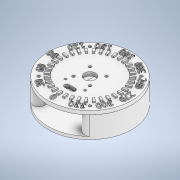
# Autodesk Inventor part: dual_motor_testbed_cover
Saved by Autodesk Inventor 2022.2 (Build 262287000, 287)
## iProperties
Created: 2018-11-22
Part Number: dual_motor_testbed_cover
Material: Generic
Document SubType Name: Modeling
Designer: Jochen
Density: 1 g/cm^3
Appearance: Default
Sending System: SolidWorks 2017
Last Author: Felix
Last Saved: 2021-02-24
Author: Jochen
Autodesk Inventor part; units mm, degrees
(part 1 of 2)
ref_plane "YZ Plane" through (0, 0, 0) normal (1, 0, 0) x (0, 1, 0)
ref_plane "XZ Plane" through (0, 0, 0) normal (0, 1, 0) x (-1, 0, 0)
ref_plane "XY Plane" through (0, 0, 0) normal (0, 0, 1) x (1, 0, 0)
sketch "Sketch1" plane through (0, 0, 0) normal (0, 1, 0) x (-1, 0, 0)
  line L0 (0, -76.3335) -> (0, 76.0077) construction
  line L1 (124.8346, 0) -> (-26.138, 0) construction
  circle A0 centre (50, 0) radius 6
  circle A1 centre (50, 0) radius 12.5 construction
  line L2 (46.5, 21.5) -> (53.5, 21.5)
  line L3 (46.5, 19) -> (53.5, 19)
  line L4 (53.5, 24) -> (46.5, 24)
  arc A2 (46.5, 24) -> (46.5, 19) centre (46.5, 21.5) ccw
  arc A3 (53.5, 19) -> (53.5, 24) centre (53.5, 21.5) ccw
  circle A4 centre (60.48, 15.75) radius 1.25
  circle A5 centre (39.52, 15.75) radius 1.25
  circle A6 centre (58.8388, 8.8388) radius 1.5
  circle A7 centre (58.8388, -8.8388) radius 1.5
  circle A8 centre (41.1612, -8.8388) radius 1.5
  circle A9 centre (41.1612, 8.8388) radius 1.5
  line L5 (58.8388, 8.8388) -> (41.1612, 8.8388) construction
  line L6 (41.1612, 8.8388) -> (41.1612, -8.8388) construction
  line L7 (41.1612, -8.8388) -> (58.8388, -8.8388) construction
  line L8 (58.8388, -8.8388) -> (58.8388, 8.8388) construction
  line L9 (50, 8.8388) -> (50, -8.8388) construction
  line L10 (51, 35) -> (49, 35)
  line L11 (49, 35) -> (49, 30)
  line L12 (49, 30) -> (51, 30)
  line L13 (51, 30) -> (51, 35)
  line L14 (85.5155, 3.449) -> (91.318, 3.449) construction
  line L15 (91.318, 3.449) -> (91.318, 5.2094) construction
  line L16 (91.318, 5.2094) -> (85.5155, 5.2094) construction
  line L17 (85.5155, 5.2094) -> (85.5155, 3.449) construction
  line L18 (43.3702, -36.2504) -> (56.0342, -36.2504) construction
  line L19 (56.0342, -36.2504) -> (56.0342, -42.8053) construction
  line L20 (56.0342, -42.8053) -> (43.3702, -42.8053) construction
  line L21 (43.3702, -42.8053) -> (43.3702, -36.2504) construction
  line L22 (9.6343, 14.1663) -> (13.2809, 21.7068) construction
  line L23 (13.2809, 21.7068) -> (20.1891, 18.366) construction
  line L24 (20.1891, 18.366) -> (16.5425, 10.8255) construction
  line L25 (16.5425, 10.8255) -> (9.6343, 14.1663) construction
  line L26 (65, 35.5829) -> (65, 35.8735) construction
  line L27 (52.3586, 36.3581) -> (47.6414, 36.3581) construction
  line L28 (47.6414, 36.3581) -> (47.6414, 35) construction
  line L29 (47.6414, 35) -> (52.3586, 35) construction
  line L30 (52.3586, 35) -> (52.3586, 36.3581) construction
  line L31 (45.7754, 29.7179) -> (44.9071, 34.6419)
  line L32 (44.9071, 34.6419) -> (42.9375, 34.2946)
  line L33 (42.9375, 34.2946) -> (43.8057, 29.3706)
  line L34 (43.8057, 29.3706) -> (45.7754, 29.7179)
  line L35 (40.6791, 28.5328) -> (38.969, 33.2313)
  line L36 (38.969, 33.2313) -> (37.0896, 32.5472)
  line L37 (37.0896, 32.5472) -> (38.7997, 27.8488)
  line L38 (38.7997, 27.8488) -> (40.6791, 28.5328)
  line L39 (35.866, 26.4808) -> (33.366, 30.8109)
  line L40 (33.366, 30.8109) -> (31.634, 29.8109)
  line L41 (31.634, 29.8109) -> (34.134, 25.4808)
  line L42 (34.134, 25.4808) -> (35.866, 26.4808)
  line L43 (31.4824, 23.6241) -> (28.2685, 27.4543)
  line L44 (28.2685, 27.4543) -> (26.7364, 26.1688)
  line L45 (26.7364, 26.1688) -> (29.9503, 22.3385)
  line L46 (29.9503, 22.3385) -> (31.4824, 23.6241)
  line L47 (27.6615, 20.0497) -> (23.8312, 23.2636)
  line L48 (23.8312, 23.2636) -> (22.5457, 21.7315)
  line L49 (22.5457, 21.7315) -> (26.3759, 18.5176)
  line L50 (26.3759, 18.5176) -> (27.6615, 20.0497)
  line L51 (24.5192, 15.866) -> (20.1891, 18.366)
  line L52 (20.1891, 18.366) -> (19.1891, 16.634)
  line L53 (19.1891, 16.634) -> (23.5192, 14.134)
  line L54 (23.5192, 14.134) -> (24.5192, 15.866)
  line L55 (22.1512, 11.2003) -> (17.4528, 12.9104)
  line L56 (17.4528, 12.9104) -> (16.7687, 11.031)
  line L57 (16.7687, 11.031) -> (21.4672, 9.3209)
  line L58 (21.4672, 9.3209) -> (22.1512, 11.2003)
  line L59 (20.6294, 6.1943) -> (15.7054, 7.0625)
  line L60 (15.7054, 7.0625) -> (15.3581, 5.0929)
  line L61 (15.3581, 5.0929) -> (20.2821, 4.2246)
  line L62 (20.2821, 4.2246) -> (20.6294, 6.1943)
  line L63 (20, 1) -> (15, 1)
  line L64 (15, 1) -> (15, -1)
  line L65 (15, -1) -> (20, -1)
  line L66 (20, -1) -> (20, 1)
  line L67 (20.2821, -4.2246) -> (15.3581, -5.0929)
  line L68 (15.3581, -5.0929) -> (15.7054, -7.0625)
  line L69 (15.7054, -7.0625) -> (20.6294, -6.1943)
  line L70 (20.6294, -6.1943) -> (20.2821, -4.2246)
  line L71 (21.4672, -9.3209) -> (16.7687, -11.031)
  line L72 (16.7687, -11.031) -> (17.4528, -12.9104)
  line L73 (17.4528, -12.9104) -> (22.1512, -11.2003)
  line L74 (22.1512, -11.2003) -> (21.4672, -9.3209)
  line L75 (23.5192, -14.134) -> (19.1891, -16.634)
  line L76 (19.1891, -16.634) -> (20.1891, -18.366)
  line L77 (20.1891, -18.366) -> (24.5192, -15.866)
  line L78 (24.5192, -15.866) -> (23.5192, -14.134)
  line L79 (26.3759, -18.5176) -> (22.5457, -21.7315)
  line L80 (22.5457, -21.7315) -> (23.8312, -23.2636)
  line L81 (23.8312, -23.2636) -> (27.6615, -20.0497)
  line L82 (27.6615, -20.0497) -> (26.3759, -18.5176)
  line L83 (29.9503, -22.3385) -> (26.7364, -26.1688)
  line L84 (26.7364, -26.1688) -> (28.2685, -27.4543)
  line L85 (28.2685, -27.4543) -> (31.4824, -23.6241)
  line L86 (31.4824, -23.6241) -> (29.9503, -22.3385)
  line L87 (34.134, -25.4808) -> (31.634, -29.8109)
  line L88 (31.634, -29.8109) -> (33.366, -30.8109)
  line L89 (33.366, -30.8109) -> (35.866, -26.4808)
  line L90 (35.866, -26.4808) -> (34.134, -25.4808)
  line L91 (38.7997, -27.8488) -> (37.0896, -32.5472)
  line L92 (37.0896, -32.5472) -> (38.969, -33.2313)
  line L93 (38.969, -33.2313) -> (40.6791, -28.5328)
  line L94 (40.6791, -28.5328) -> (38.7997, -27.8488)
  line L95 (43.8057, -29.3706) -> (42.9375, -34.2946)
  line L96 (42.9375, -34.2946) -> (44.9071, -34.6419)
  line L97 (44.9071, -34.6419) -> (45.7754, -29.7179)
  line L98 (45.7754, -29.7179) -> (43.8057, -29.3706)
  line L99 (49, -30) -> (49, -35)
  line L100 (49, -35) -> (51, -35)
  line L101 (51, -35) -> (51, -30)
  line L102 (51, -30) -> (49, -30)
  line L103 (54.2246, -29.7179) -> (55.0929, -34.6419)
  line L104 (55.0929, -34.6419) -> (57.0625, -34.2946)
  line L105 (57.0625, -34.2946) -> (56.1943, -29.3706)
  line L106 (56.1943, -29.3706) -> (54.2246, -29.7179)
  line L107 (59.3209, -28.5328) -> (61.031, -33.2313)
  line L108 (61.031, -33.2313) -> (62.9104, -32.5472)
  line L109 (62.9104, -32.5472) -> (61.2003, -27.8488)
  line L110 (61.2003, -27.8488) -> (59.3209, -28.5328)
  line L111 (64.134, -26.4808) -> (66.634, -30.8109)
  line L112 (66.634, -30.8109) -> (68.366, -29.8109)
  line L113 (68.366, -29.8109) -> (65.866, -25.4808)
  line L114 (65.866, -25.4808) -> (64.134, -26.4808)
  line L115 (68.5176, -23.6241) -> (71.7315, -27.4543)
  line L116 (71.7315, -27.4543) -> (73.2636, -26.1688)
  line L117 (73.2636, -26.1688) -> (70.0497, -22.3385)
  line L118 (70.0497, -22.3385) -> (68.5176, -23.6241)
  line L119 (72.3385, -20.0497) -> (76.1688, -23.2636)
  line L120 (76.1688, -23.2636) -> (77.4543, -21.7315)
  line L121 (77.4543, -21.7315) -> (73.6241, -18.5176)
  line L122 (73.6241, -18.5176) -> (72.3385, -20.0497)
  line L123 (75.4808, -15.866) -> (79.8109, -18.366)
  line L124 (79.8109, -18.366) -> (80.8109, -16.634)
  line L125 (80.8109, -16.634) -> (76.4808, -14.134)
  line L126 (76.4808, -14.134) -> (75.4808, -15.866)
  line L127 (77.8488, -11.2003) -> (82.5472, -12.9104)
  line L128 (82.5472, -12.9104) -> (83.2313, -11.031)
  line L129 (83.2313, -11.031) -> (78.5328, -9.3209)
  line L130 (78.5328, -9.3209) -> (77.8488, -11.2003)
  line L131 (79.3706, -6.1943) -> (84.2946, -7.0625)
  line L132 (84.2946, -7.0625) -> (84.6419, -5.0929)
  line L133 (84.6419, -5.0929) -> (79.7179, -4.2246)
  line L134 (79.7179, -4.2246) -> (79.3706, -6.1943)
  line L135 (80, -1) -> (85, -1)
  line L136 (85, -1) -> (85, 1)
  line L137 (85, 1) -> (80, 1)
  line L138 (80, 1) -> (80, -1)
  line L139 (79.7179, 4.2246) -> (84.6419, 5.0929)
  line L140 (84.6419, 5.0929) -> (84.2946, 7.0625)
  line L141 (84.2946, 7.0625) -> (79.3706, 6.1943)
  line L142 (79.3706, 6.1943) -> (79.7179, 4.2246)
  line L143 (78.5328, 9.3209) -> (83.2313, 11.031)
  line L144 (83.2313, 11.031) -> (82.5472, 12.9104)
  line L145 (82.5472, 12.9104) -> (77.8488, 11.2003)
  line L146 (77.8488, 11.2003) -> (78.5328, 9.3209)
  line L147 (76.4808, 14.134) -> (80.8109, 16.634)
  line L148 (80.8109, 16.634) -> (79.8109, 18.366)
  line L149 (79.8109, 18.366) -> (75.4808, 15.866)
  line L150 (75.4808, 15.866) -> (76.4808, 14.134)
  line L151 (73.6241, 18.5176) -> (77.4543, 21.7315)
  line L152 (77.4543, 21.7315) -> (76.1688, 23.2636)
  line L153 (76.1688, 23.2636) -> (72.3385, 20.0497)
  line L154 (72.3385, 20.0497) -> (73.6241, 18.5176)
  line L155 (70.0497, 22.3385) -> (73.2636, 26.1688)
  line L156 (73.2636, 26.1688) -> (71.7315, 27.4543)
  line L157 (71.7315, 27.4543) -> (68.5176, 23.6241)
  line L158 (68.5176, 23.6241) -> (70.0497, 22.3385)
  line L159 (65.866, 25.4808) -> (68.366, 29.8109)
  line L160 (68.366, 29.8109) -> (66.634, 30.8109)
  line L161 (66.634, 30.8109) -> (64.134, 26.4808)
  line L162 (64.134, 26.4808) -> (65.866, 25.4808)
  line L163 (61.2003, 27.8488) -> (62.9104, 32.5472)
  line L164 (62.9104, 32.5472) -> (61.031, 33.2313)
  line L165 (61.031, 33.2313) -> (59.3209, 28.5328)
  line L166 (59.3209, 28.5328) -> (61.2003, 27.8488)
  line L167 (56.1943, 29.3706) -> (57.0625, 34.2946)
  line L168 (57.0625, 34.2946) -> (55.0929, 34.6419)
  line L169 (55.0929, 34.6419) -> (54.2246, 29.7179)
  line L170 (54.2246, 29.7179) -> (56.1943, 29.3706)
  arc A10 (95, 0) -> (10.2941, 21.1765) centre (50, 0) ccw
  arc A11 (10.2941, 21.1765) -> (95, 0) centre (50, 0) ccw
  circle A12 centre (77.5, 27.5) radius 1.5
  circle A13 centre (77.5, -27.5) radius 1.5
  circle A14 centre (22.5, -27.5) radius 1.5
  circle A15 centre (22.5, 27.5) radius 1.5
  line L171 (77.5, 27.5) -> (22.5, 27.5) construction
  line L172 (22.5, 27.5) -> (22.5, -27.5) construction
  line L173 (22.5, -27.5) -> (77.5, -27.5) construction
  line L174 (77.5, -27.5) -> (77.5, 27.5) construction
  line L175 (71.3909, 27.5) -> (71.3909, -27.5)
  arc A16 (71.3909, -27.5) -> (81.8198, -31.8198) centre (77.5, -27.5) ccw
  arc A17 (18.1802, -31.8198) -> (28.6091, -27.5) centre (22.5, -27.5) ccw
  arc A18 (81.8198, 31.8198) -> (71.3909, 27.5) centre (77.5, 27.5) ccw
  arc A19 (28.6091, 27.5) -> (18.1802, 31.8198) centre (22.5, 27.5) ccw
  line L176 (28.6091, 27.5) -> (28.6091, -27.5)
  line L177 (7.333, -7.0802) -> (7.333, 0) construction
  line L178 (7.333, 0) -> (17.5306, 0) construction
  line L179 (17.5306, 0) -> (17.5306, -7.0802) construction
  line L180 (17.5306, -7.0802) -> (7.333, -7.0802) construction
  line L181 (22.3605, 33.283) -> (34.2819, 40.1658) construction
  line L182 (34.2819, 40.1658) -> (31.501, 44.9824) construction
  line L183 (31.501, 44.9824) -> (19.5797, 38.0996) construction
  line L184 (19.5797, 38.0996) -> (22.3605, 33.283) construction
  line L185 (16.4835, -27.645) -> (12.2955, -20.3911) construction
  line L186 (12.2955, -20.3911) -> (18.941, -16.5543) construction
  line L187 (18.941, -16.5543) -> (23.129, -23.8082) construction
  line L188 (23.129, -23.8082) -> (16.4835, -27.645) construction
  line L189 (25.9985, -27.8884) -> (33.1783, -32.0337) construction
  line L190 (33.1783, -32.0337) -> (25.8889, -44.6591) construction
  line L191 (25.8889, -44.6591) -> (18.7092, -40.5139) construction
  line L192 (18.7092, -40.5139) -> (25.9985, -27.8884) construction
  line L193 (69.3835, -47.2114) -> (62.0942, -34.5859) construction
  line L194 (62.0942, -34.5859) -> (69.2739, -30.4407) construction
  line L195 (69.2739, -30.4407) -> (76.5632, -43.0661) construction
  line L196 (76.5632, -43.0661) -> (69.3835, -47.2114) construction
  line L197 (90.9137, -31.4796) -> (78.2883, -24.1903) construction
  line L198 (78.2883, -24.1903) -> (82.4335, -17.0105) construction
  line L199 (82.4335, -17.0105) -> (95.059, -24.2998) construction
  line L200 (95.059, -24.2998) -> (90.9137, -31.4796) construction
  line L201 (70.6585, 43.5756) -> (67.8777, 38.759) construction
  line L202 (67.8777, 38.759) -> (79.799, 31.8762) construction
  line L203 (79.799, 31.8762) -> (82.5798, 36.6928) construction
  line L204 (82.5798, 36.6928) -> (70.6585, 43.5756) construction
  line L205 (89.2101, 27.3822) -> (84.3935, 24.6014) construction
  line L206 (84.3935, 24.6014) -> (91.2763, 12.68) construction
  line L207 (91.2763, 12.68) -> (96.0929, 15.4608) construction
  line L208 (96.0929, 15.4608) -> (89.2101, 27.3822) construction
  spline S0 degree 2 poles (11.181, 15.741) (11.0842, 15.5407) (10.9905, 15.0973) (10.9737, 14.8694) knots 0 0 0 1 2 2 2
  spline S1 degree 2 poles (10.9737, 14.8694) (10.9632, 14.6548) (10.9965, 14.3147) (11.0182, 14.1779) knots 0 0 0 1 2 2 2
  line L209 (11.0182, 14.1779) -> (10.9966, 14.1334)
  line L210 (10.9966, 14.1334) -> (10.2179, 14.5101)
  spline S2 degree 2 poles (10.2179, 14.5101) (10.205, 14.8128) (10.394, 15.7372) (10.5726, 16.1066) knots 0 0 0 1 2 2 2
  spline S3 degree 2 poles (10.5726, 16.1066) (10.7534, 16.4804) (11.1737, 16.9635) (11.4437, 17.113) knots 0 0 0 1 2 2 2
  spline S4 degree 2 poles (11.4437, 17.113) (11.7335, 17.2694) (12.3569, 17.2754) (12.6951, 17.1118) knots 0 0 0 1 2 2 2
  spline S5 degree 2 poles (12.6951, 17.1118) (13.149, 16.8923) (13.5459, 15.9645) (13.4326, 15.5032) knots 0 0 0 1 2 2 2
  line L211 (13.4326, 15.5032) -> (13.486, 15.4774)
  spline S6 degree 2 poles (13.486, 15.4774) (13.6056, 15.6337) (13.9573, 15.9523) (14.1993, 16.0439) knots 0 0 0 1 2 2 2
  spline S7 degree 2 poles (14.1993, 16.0439) (14.4369, 16.1377) (15.0386, 16.1103) (15.399, 15.9359) knots 0 0 0 1 2 2 2
  spline S8 degree 2 poles (15.399, 15.9359) (15.7684, 15.7573) (16.2732, 15.2002) (16.4016, 14.8526) knots 0 0 0 1 2 2 2
  spline S9 degree 2 poles (16.4016, 14.8526) (16.5346, 14.4917) (16.4634, 13.686) (16.2547, 13.2544) knots 0 0 0 1 2 2 2
  spline S10 degree 2 poles (16.2547, 13.2544) (16.0545, 12.8405) (15.4626, 12.1274) (15.1912, 11.9182) knots 0 0 0 1 2 2 2
  line L212 (15.1912, 11.9182) -> (14.4124, 12.2948)
  line L213 (14.4124, 12.2948) -> (14.4382, 12.3482)
  spline S11 degree 2 poles (14.4382, 12.3482) (14.7193, 12.4979) (15.4096, 13.1305) (15.5968, 13.5176) knots 0 0 0 1 2 2 2
  spline S12 degree 2 poles (15.5968, 13.5176) (15.7065, 13.7446) (15.7837, 14.2674) (15.6922, 14.4983) knots 0 0 0 1 2 2 2
  spline S13 degree 2 poles (15.6922, 14.4983) (15.5985, 14.7248) (15.2822, 15.0699) (14.9841, 15.2141) knots 0 0 0 1 2 2 2
  spline S14 degree 2 poles (14.9841, 15.2141) (14.6859, 15.3583) (14.2148, 15.372) (14.0282, 15.2701) knots 0 0 0 1 2 2 2
  spline S15 degree 2 poles (14.0282, 15.2701) (13.8417, 15.1681) (13.5527, 14.7862) (13.4321, 14.537) knots 0 0 0 1 2 2 2
  line L214 (13.4321, 14.537) -> (13.2815, 14.2255)
  line L215 (13.2815, 14.2255) -> (12.6718, 14.5203)
  line L216 (12.6718, 14.5203) -> (12.7902, 14.7651)
  spline S16 degree 2 poles (12.7902, 14.7651) (13.0291, 15.2591) (12.8586, 16.1102) (12.4092, 16.3276) knots 0 0 0 1 2 2 2
  spline S17 degree 2 poles (12.4092, 16.3276) (12.2, 16.4287) (11.8244, 16.4127) (11.673, 16.3267) knots 0 0 0 1 2 2 2
  spline S18 degree 2 poles (11.673, 16.3267) (11.5128, 16.234) (11.2736, 15.9323) (11.181, 15.741) knots 0 0 0 1 2 2 2
  spline S19 degree 2 poles (16.3352, 20.7216) (17.8126, 20.0071) (18.7813, 18.4789) (18.3487, 17.5844) knots 0 0 0 1 2 2 2
  spline S20 degree 2 poles (18.3487, 17.5844) (17.9097, 16.6766) (16.0879, 16.5088) (14.6416, 17.2083) knots 0 0 0 1 2 2 2
  spline S21 degree 2 poles (14.6416, 17.2083) (13.1552, 17.9271) (12.1955, 19.451) (12.6302, 20.3499) knots 0 0 0 1 2 2 2
  spline S22 degree 2 poles (12.6302, 20.3499) (13.0671, 21.2533) (14.9022, 21.4146) (16.3352, 20.7216) knots 0 0 0 1 2 2 2
  spline S23 degree 2 poles (17.5522, 18.969) (17.3324, 19.2071) (16.5388, 19.7007) (15.9736, 19.974) knots 0 0 0 1 2 2 2
  spline S24 degree 2 poles (15.9736, 19.974) (15.4084, 20.2473) (14.5332, 20.5608) (14.1991, 20.5851) knots 0 0 0 1 2 2 2
  spline S25 degree 2 poles (14.1991, 20.5851) (13.8649, 20.6094) (13.3884, 20.3621) (13.2399, 20.0551) knots 0 0 0 1 2 2 2
  spline S26 degree 2 poles (13.2399, 20.0551) (13.0914, 19.748) (13.1891, 19.2121) (13.4224, 18.9565) knots 0 0 0 1 2 2 2
  spline S27 degree 2 poles (13.4224, 18.9565) (13.649, 18.7096) (14.4647, 18.2163) (15.0032, 17.9559) knots 0 0 0 1 2 2 2
  spline S28 degree 2 poles (15.0032, 17.9559) (15.5817, 17.6761) (16.3904, 17.3728) (16.749, 17.3422) knots 0 0 0 1 2 2 2
  spline S29 degree 2 poles (16.749, 17.3422) (17.0855, 17.3113) (17.5841, 17.5588) (17.739, 17.8793) knots 0 0 0 1 2 2 2
  spline S30 degree 2 poles (17.739, 17.8793) (17.8854, 18.1819) (17.7877, 18.7178) (17.5522, 18.969) knots 0 0 0 1 2 2 2
  spline S31 degree 2 poles (18.3281, 24.8425) (19.8055, 24.128) (20.7742, 22.5998) (20.3416, 21.7053) knots 0 0 0 1 2 2 2
  spline S32 degree 2 poles (20.3416, 21.7053) (19.9026, 20.7975) (18.0808, 20.6297) (16.6345, 21.3291) knots 0 0 0 1 2 2 2
  spline S33 degree 2 poles (16.6345, 21.3291) (15.1481, 22.048) (14.1884, 23.5719) (14.6231, 24.4708) knots 0 0 0 1 2 2 2
  spline S34 degree 2 poles (14.6231, 24.4708) (15.06, 25.3742) (16.8951, 25.5355) (18.3281, 24.8425) knots 0 0 0 1 2 2 2
  spline S35 degree 2 poles (19.5451, 23.0899) (19.3253, 23.3279) (18.5317, 23.8215) (17.9665, 24.0949) knots 0 0 0 1 2 2 2
  spline S36 degree 2 poles (17.9665, 24.0949) (17.4013, 24.3682) (16.5261, 24.6816) (16.1919, 24.706) knots 0 0 0 1 2 2 2
  spline S37 degree 2 poles (16.1919, 24.706) (15.8578, 24.7303) (15.3813, 24.483) (15.2328, 24.176) knots 0 0 0 1 2 2 2
  spline S38 degree 2 poles (15.2328, 24.176) (15.0843, 23.8689) (15.182, 23.3329) (15.4153, 23.0773) knots 0 0 0 1 2 2 2
  spline S39 degree 2 poles (15.4153, 23.0773) (15.6419, 22.8305) (16.4576, 22.3372) (16.996, 22.0768) knots 0 0 0 1 2 2 2
  spline S40 degree 2 poles (16.996, 22.0768) (17.5746, 21.797) (18.3833, 21.4937) (18.7419, 21.4631) knots 0 0 0 1 2 2 2
  spline S41 degree 2 poles (18.7419, 21.4631) (19.0784, 21.4322) (19.577, 21.6797) (19.7319, 22.0001) knots 0 0 0 1 2 2 2
  spline S42 degree 2 poles (19.7319, 22.0001) (19.8783, 22.3028) (19.7805, 22.8387) (19.5451, 23.0899) knots 0 0 0 1 2 2 2
  line L217 (47.2705, -42.4888) -> (44.2946, -42.4888)
  line L218 (44.2946, -42.4888) -> (44.2946, -41.866)
  line L219 (44.2946, -41.866) -> (45.4019, -41.866)
  line L220 (45.4019, -41.866) -> (45.4019, -37.7779)
  line L221 (45.4019, -37.7779) -> (44.2946, -37.7779)
  line L222 (44.2946, -37.7779) -> (44.2946, -37.2193)
  spline S43 degree 2 poles (44.2946, -37.2193) (44.9224, -37.2193) (45.5156, -36.8634) (45.5552, -36.3691) knots 0 0 0 1 2 2 2
  line L223 (45.5552, -36.3691) -> (46.1879, -36.3691)
  line L224 (46.1879, -36.3691) -> (46.1879, -41.866)
  line L225 (46.1879, -41.866) -> (47.2705, -41.866)
  line L226 (47.2705, -41.866) -> (47.2705, -42.4888)
  spline S44 degree 2 poles (50.2365, -42.6272) (49.7817, -42.6272) (49.0352, -42.3554) (48.7732, -42.1033) knots 0 0 0 1 2 2 2
  spline S45 degree 2 poles (48.7732, -42.1033) (48.5162, -41.8561) (48.2493, -41.1838) (48.2493, -40.8032) knots 0 0 0 1 2 2 2
  spline S46 degree 2 poles (48.2493, -40.8032) (48.2493, -40.3089) (48.7782, -39.4784) (49.2824, -39.2312) knots 0 0 0 1 2 2 2
  line L227 (49.2824, -39.2312) -> (49.2824, -39.2065)
  spline S47 degree 2 poles (49.2824, -39.2065) (48.8326, -38.9445) (48.3976, -38.3217) (48.3976, -37.857) knots 0 0 0 1 2 2 2
  spline S48 degree 2 poles (48.3976, -37.857) (48.3976, -37.1699) (49.4356, -36.2504) (50.2365, -36.2504) knots 0 0 0 1 2 2 2
  spline S49 degree 2 poles (50.2365, -36.2504) (51.0669, -36.2504) (52.0704, -37.1204) (52.0704, -37.8026) knots 0 0 0 1 2 2 2
  spline S50 degree 2 poles (52.0704, -37.8026) (52.0704, -38.2129) (51.5909, -39.0137) (51.1411, -39.2411) knots 0 0 0 1 2 2 2
  line L228 (51.1411, -39.2411) -> (51.1411, -39.2658)
  spline S51 degree 2 poles (51.1411, -39.2658) (51.6749, -39.513) (52.2237, -40.2248) (52.2237, -40.7883) knots 0 0 0 1 2 2 2
  spline S52 degree 2 poles (52.2237, -40.7883) (52.2237, -41.5694) (51.0867, -42.6272) (50.2365, -42.6272) knots 0 0 0 1 2 2 2
  spline S53 degree 2 poles (51.3833, -40.8674) (51.3833, -40.4918) (51.0867, -40.0469) (50.6665, -39.8195) knots 0 0 0 1 2 2 2
  spline S54 degree 2 poles (50.6665, -39.8195) (50.5281, -39.7404) (50.0634, -39.5575) (49.7718, -39.4388) knots 0 0 0 1 2 2 2
  spline S55 degree 2 poles (49.7718, -39.4388) (49.4356, -39.6613) (49.0748, -40.3237) (49.0748, -40.7439) knots 0 0 0 1 2 2 2
  spline S56 degree 2 poles (49.0748, -40.7439) (49.0748, -41.2975) (49.7421, -42.0192) (50.2463, -42.0192) knots 0 0 0 1 2 2 2
  spline S57 degree 2 poles (50.2463, -42.0192) (50.7604, -42.0192) (51.3833, -41.4013) (51.3833, -40.8674) knots 0 0 0 1 2 2 2
  spline S58 degree 2 poles (51.2696, -37.8125) (51.2696, -37.4022) (50.7209, -36.8535) (50.2315, -36.8535) knots 0 0 0 1 2 2 2
  spline S59 degree 2 poles (50.2315, -36.8535) (49.7866, -36.8535) (49.2181, -37.3429) (49.2181, -37.7631) knots 0 0 0 1 2 2 2
  spline S60 degree 2 poles (49.2181, -37.7631) (49.2181, -38.0646) (49.5098, -38.4848) (49.8014, -38.6529) knots 0 0 0 1 2 2 2
  spline S61 degree 2 poles (49.8014, -38.6529) (49.925, -38.7221) (50.449, -38.9643) (50.6616, -39.0335) knots 0 0 0 1 2 2 2
  spline S62 degree 2 poles (50.6616, -39.0335) (51.0175, -38.7616) (51.2696, -38.1832) (51.2696, -37.8125) knots 0 0 0 1 2 2 2
  spline S63 degree 2 poles (56.7665, -39.4388) (56.7665, -41.08) (55.8125, -42.6174) (54.8189, -42.6174) knots 0 0 0 1 2 2 2
  spline S64 degree 2 poles (54.8189, -42.6174) (53.8104, -42.6174) (52.8663, -41.0503) (52.8663, -39.4438) knots 0 0 0 1 2 2 2
  spline S65 degree 2 poles (52.8663, -39.4438) (52.8663, -37.7927) (53.8203, -36.2653) (54.8189, -36.2653) knots 0 0 0 1 2 2 2
  spline S66 degree 2 poles (54.8189, -36.2653) (55.8224, -36.2653) (56.7665, -37.8471) (56.7665, -39.4388) knots 0 0 0 1 2 2 2
  spline S67 degree 2 poles (55.7185, -41.2975) (55.8372, -40.996) (55.9361, -40.0666) (55.9361, -39.4388) knots 0 0 0 1 2 2 2
  spline S68 degree 2 poles (55.9361, -39.4388) (55.9361, -38.811) (55.8372, -37.8866) (55.7136, -37.5752) knots 0 0 0 1 2 2 2
  spline S69 degree 2 poles (55.7136, -37.5752) (55.59, -37.2638) (55.16, -36.9425) (54.8189, -36.9425) knots 0 0 0 1 2 2 2
  spline S70 degree 2 poles (54.8189, -36.9425) (54.4778, -36.9425) (54.0378, -37.2638) (53.9093, -37.5851) knots 0 0 0 1 2 2 2
  spline S71 degree 2 poles (53.9093, -37.5851) (53.7857, -37.8965) (53.6967, -38.8456) (53.6967, -39.4438) knots 0 0 0 1 2 2 2
  spline S72 degree 2 poles (53.6967, -39.4438) (53.6967, -40.0864) (53.7758, -40.9465) (53.9044, -41.2827) knots 0 0 0 1 2 2 2
  spline S73 degree 2 poles (53.9044, -41.2827) (54.023, -41.599) (54.463, -41.9401) (54.8189, -41.9401) knots 0 0 0 1 2 2 2
  spline S74 degree 2 poles (54.8189, -41.9401) (55.155, -41.9401) (55.595, -41.6188) (55.7185, -41.2975) knots 0 0 0 1 2 2 2
  spline S75 degree 2 poles (85.7923, 1.3431) (85.7923, 1.8128) (86.0988, 2.5938) (86.3658, 2.8756) knots 0 0 0 1 2 2 2
  spline S76 degree 2 poles (86.3658, 2.8756) (86.6179, 3.1474) (87.3544, 3.449) (87.7301, 3.449) knots 0 0 0 1 2 2 2
  spline S77 degree 2 poles (87.7301, 3.449) (88.1503, 3.449) (88.8325, 3.1672) (89.0846, 2.9003) knots 0 0 0 1 2 2 2
  spline S78 degree 2 poles (89.0846, 2.9003) (89.4009, 2.5641) (89.747, 1.4766) (89.747, 0.6412) knots 0 0 0 1 2 2 2
  spline S79 degree 2 poles (89.747, 0.6412) (89.747, -0.1151) (89.4059, -1.4696) (89.0747, -1.9194) knots 0 0 0 1 2 2 2
  spline S80 degree 2 poles (89.0747, -1.9194) (88.7237, -2.394) (87.735, -2.8932) (87.0133, -2.8932) knots 0 0 0 1 2 2 2
  spline S81 degree 2 poles (87.0133, -2.8932) (86.8502, -2.8932) (86.4795, -2.8586) (86.3213, -2.8092) knots 0 0 0 1 2 2 2
  line L229 (86.3213, -2.8092) -> (86.3213, -2.0232)
  line L230 (86.3213, -2.0232) -> (86.3608, -2.0232)
  spline S82 degree 2 poles (86.3608, -2.0232) (86.4646, -2.0825) (86.8996, -2.1864) (87.1221, -2.1864) knots 0 0 0 1 2 2 2
  spline S83 degree 2 poles (87.1221, -2.1864) (87.9229, -2.1864) (88.8374, -1.1285) (88.9017, -0.1497) knots 0 0 0 1 2 2 2
  spline S84 degree 2 poles (88.9017, -0.1497) (88.5754, -0.3722) (87.9822, -0.5749) (87.6312, -0.5749) knots 0 0 0 1 2 2 2
  spline S85 degree 2 poles (87.6312, -0.5749) (87.2951, -0.5749) (86.7365, -0.4266) (86.4547, -0.214) knots 0 0 0 1 2 2 2
  spline S86 degree 2 poles (86.4547, -0.214) (86.1285, 0.0381) (85.7923, 0.8043) (85.7923, 1.3431) knots 0 0 0 1 2 2 2
  spline S87 degree 2 poles (88.9214, 0.8241) (88.9214, 1.442) (88.694, 2.223) (88.4914, 2.4356) knots 0 0 0 1 2 2 2
  spline S88 degree 2 poles (88.4914, 2.4356) (88.3134, 2.6333) (87.9427, 2.7816) (87.7252, 2.7816) knots 0 0 0 1 2 2 2
  spline S89 degree 2 poles (87.7252, 2.7816) (87.2209, 2.7816) (86.6228, 2.0599) (86.6228, 1.3777) knots 0 0 0 1 2 2 2
  spline S90 degree 2 poles (86.6228, 1.3777) (86.6228, 0.9922) (86.8205, 0.4929) (87.038, 0.3149) knots 0 0 0 1 2 2 2
  spline S91 degree 2 poles (87.038, 0.3149) (87.1962, 0.1864) (87.5867, 0.1024) (87.8141, 0.1024) knots 0 0 0 1 2 2 2
  spline S92 degree 2 poles (87.8141, 0.1024) (88.0761, 0.1024) (88.6792, 0.2853) (88.9066, 0.4385) knots 0 0 0 1 2 2 2
  spline S93 degree 2 poles (88.9066, 0.4385) (88.9115, 0.4978) (88.9214, 0.7005) (88.9214, 0.8241) knots 0 0 0 1 2 2 2
  spline S94 degree 2 poles (94.3343, 0.2754) (94.3343, -1.3658) (93.3803, -2.9031) (92.3867, -2.9031) knots 0 0 0 1 2 2 2
  spline S95 degree 2 poles (92.3867, -2.9031) (91.3782, -2.9031) (90.4341, -1.3361) (90.4341, 0.2704) knots 0 0 0 1 2 2 2
  spline S96 degree 2 poles (90.4341, 0.2704) (90.4341, 1.9215) (91.3881, 3.449) (92.3867, 3.449) knots 0 0 0 1 2 2 2
  spline S97 degree 2 poles (92.3867, 3.449) (93.3902, 3.449) (94.3343, 1.8671) (94.3343, 0.2754) knots 0 0 0 1 2 2 2
  spline S98 degree 2 poles (93.2863, -1.5833) (93.405, -1.2817) (93.5038, -0.3524) (93.5038, 0.2754) knots 0 0 0 1 2 2 2
  spline S99 degree 2 poles (93.5038, 0.2754) (93.5038, 0.9032) (93.405, 1.8276) (93.2814, 2.139) knots 0 0 0 1 2 2 2
  spline S100 degree 2 poles (93.2814, 2.139) (93.1578, 2.4504) (92.7278, 2.7717) (92.3867, 2.7717) knots 0 0 0 1 2 2 2
  spline S101 degree 2 poles (92.3867, 2.7717) (92.0456, 2.7717) (91.6056, 2.4504) (91.4771, 2.1291) knots 0 0 0 1 2 2 2
  spline S102 degree 2 poles (91.4771, 2.1291) (91.3535, 1.8177) (91.2645, 0.8686) (91.2645, 0.2704) knots 0 0 0 1 2 2 2
  spline S103 degree 2 poles (91.2645, 0.2704) (91.2645, -0.3722) (91.3436, -1.2323) (91.4722, -1.5684) knots 0 0 0 1 2 2 2
  spline S104 degree 2 poles (91.4722, -1.5684) (91.5908, -1.8848) (92.0308, -2.2259) (92.3867, -2.2259) knots 0 0 0 1 2 2 2
  spline S105 degree 2 poles (92.3867, -2.2259) (92.7228, -2.2259) (93.1628, -1.9046) (93.2863, -1.5833) knots 0 0 0 1 2 2 2
  spline S106 degree 2 poles (48.1173, 39.5317) (48.1173, 41.1729) (49.0714, 42.7103) (50.065, 42.7103) knots 0 0 0 1 2 2 2
  spline S107 degree 2 poles (50.065, 42.7103) (51.0734, 42.7103) (52.0175, 41.1432) (52.0175, 39.5367) knots 0 0 0 1 2 2 2
  spline S108 degree 2 poles (52.0175, 39.5367) (52.0175, 37.8856) (51.0635, 36.3581) (50.065, 36.3581) knots 0 0 0 1 2 2 2
  spline S109 degree 2 poles (50.065, 36.3581) (49.0615, 36.3581) (48.1173, 37.94) (48.1173, 39.5317) knots 0 0 0 1 2 2 2
  spline S110 degree 2 poles (49.1653, 41.3904) (49.0466, 41.0889) (48.9478, 40.1595) (48.9478, 39.5317) knots 0 0 0 1 2 2 2
  spline S111 degree 2 poles (48.9478, 39.5317) (48.9478, 38.9039) (49.0466, 37.9795) (49.1702, 37.6681) knots 0 0 0 1 2 2 2
  spline S112 degree 2 poles (49.1702, 37.6681) (49.2938, 37.3567) (49.7239, 37.0354) (50.065, 37.0354) knots 0 0 0 1 2 2 2
  spline S113 degree 2 poles (50.065, 37.0354) (50.406, 37.0354) (50.846, 37.3567) (50.9745, 37.678) knots 0 0 0 1 2 2 2
  spline S114 degree 2 poles (50.9745, 37.678) (51.0981, 37.9894) (51.1871, 38.9385) (51.1871, 39.5367) knots 0 0 0 1 2 2 2
  spline S115 degree 2 poles (51.1871, 39.5367) (51.1871, 40.1793) (51.108, 41.0394) (50.9795, 41.3756) knots 0 0 0 1 2 2 2
  spline S116 degree 2 poles (50.9795, 41.3756) (50.8608, 41.6919) (50.4209, 42.033) (50.065, 42.033) knots 0 0 0 1 2 2 2
  spline S117 degree 2 poles (50.065, 42.033) (49.7288, 42.033) (49.2889, 41.7117) (49.1653, 41.3904) knots 0 0 0 1 2 2 2
  spline S118 degree 2 poles (24.5248, 33.7164) (24.3322, 33.6051) (24.0056, 33.291) (23.8635, 33.1119) knots 0 0 0 1 2 2 2
  spline S119 degree 2 poles (23.8635, 33.1119) (23.7343, 32.9403) (23.5707, 32.6403) (23.5118, 32.515) knots 0 0 0 1 2 2 2
  line L231 (23.5118, 32.515) -> (23.469, 32.4903)
  line L232 (23.469, 32.4903) -> (23.0364, 33.2394)
  spline S120 degree 2 poles (23.0364, 33.2394) (23.1959, 33.4971) (23.8717, 34.1555) (24.2271, 34.3607) knots 0 0 0 1 2 2 2
  spline S121 degree 2 poles (24.2271, 34.3607) (24.5867, 34.5683) (25.2058, 34.7317) (25.5131, 34.7036) knots 0 0 0 1 2 2 2
  spline S122 degree 2 poles (25.5131, 34.7036) (25.8407, 34.6701) (26.3597, 34.3248) (26.5476, 33.9994) knots 0 0 0 1 2 2 2
  spline S123 degree 2 poles (26.5476, 33.9994) (26.7997, 33.5628) (26.6067, 32.5723) (26.2537, 32.2543) knots 0 0 0 1 2 2 2
  line L233 (26.2537, 32.2543) -> (26.2833, 32.203)
  spline S124 degree 2 poles (26.2833, 32.203) (26.4701, 32.2651) (26.9401, 32.331) (27.1917, 32.2708) knots 0 0 0 1 2 2 2
  spline S125 degree 2 poles (27.1917, 32.2708) (27.4409, 32.2149) (27.9232, 31.854) (28.1234, 31.5073) knots 0 0 0 1 2 2 2
  spline S126 degree 2 poles (28.1234, 31.5073) (28.3286, 31.152) (28.433, 30.4075) (28.3439, 30.0478) knots 0 0 0 1 2 2 2
  spline S127 degree 2 poles (28.3439, 30.0478) (28.2511, 29.6745) (27.7395, 29.0481) (27.3242, 28.8083) knots 0 0 0 1 2 2 2
  spline S128 degree 2 poles (27.3242, 28.8083) (26.9261, 28.5785) (26.0357, 28.3213) (25.6937, 28.3008) knots 0 0 0 1 2 2 2
  line L234 (25.6937, 28.3008) -> (25.2612, 29.0499)
  line L235 (25.2612, 29.0499) -> (25.3125, 29.0796)
  spline S129 degree 2 poles (25.3125, 29.0796) (25.6291, 29.0454) (26.5555, 29.1808) (26.928, 29.3958) knots 0 0 0 1 2 2 2
  spline S130 degree 2 poles (26.928, 29.3958) (27.1463, 29.5219) (27.5039, 29.911) (27.558, 30.1534) knots 0 0 0 1 2 2 2
  spline S131 degree 2 poles (27.558, 30.1534) (27.6078, 30.3934) (27.5401, 30.8566) (27.3745, 31.1434) knots 0 0 0 1 2 2 2
  spline S132 degree 2 poles (27.3745, 31.1434) (27.2089, 31.4302) (26.827, 31.7063) (26.6153, 31.7268) knots 0 0 0 1 2 2 2
  spline S133 degree 2 poles (26.6153, 31.7268) (26.4037, 31.7473) (25.95, 31.5939) (25.7103, 31.4555) knots 0 0 0 1 2 2 2
  line L236 (25.7103, 31.4555) -> (25.4106, 31.2824)
  line L237 (25.4106, 31.2824) -> (25.072, 31.8689)
  line L238 (25.072, 31.8689) -> (25.3075, 32.0049)
  spline S134 degree 2 poles (25.3075, 32.0049) (25.7827, 32.2792) (26.12, 33.079) (25.8704, 33.5114) knots 0 0 0 1 2 2 2
  spline S135 degree 2 poles (25.8704, 33.5114) (25.7542, 33.7126) (25.4345, 33.9105) (25.2609, 33.9244) knots 0 0 0 1 2 2 2
  spline S136 degree 2 poles (25.2609, 33.9244) (25.0763, 33.9377) (24.7089, 33.8226) (24.5248, 33.7164) knots 0 0 0 1 2 2 2
  spline S137 degree 2 poles (28.4891, 36.0051) (28.2964, 35.8939) (27.9698, 35.5797) (27.8277, 35.4007) knots 0 0 0 1 2 2 2
  spline S138 degree 2 poles (27.8277, 35.4007) (27.6985, 35.229) (27.5349, 34.9291) (27.476, 34.8037) knots 0 0 0 1 2 2 2
  line L239 (27.476, 34.8037) -> (27.4332, 34.779)
  line L240 (27.4332, 34.779) -> (27.0006, 35.5282)
  spline S139 degree 2 poles (27.0006, 35.5282) (27.1601, 35.7858) (27.8359, 36.4443) (28.1913, 36.6494) knots 0 0 0 1 2 2 2
  spline S140 degree 2 poles (28.1913, 36.6494) (28.5509, 36.857) (29.17, 37.0204) (29.4773, 36.9924) knots 0 0 0 1 2 2 2
  spline S141 degree 2 poles (29.4773, 36.9924) (29.8049, 36.9589) (30.3239, 36.6135) (30.5118, 36.2882) knots 0 0 0 1 2 2 2
  spline S142 degree 2 poles (30.5118, 36.2882) (30.7639, 35.8515) (30.5709, 34.861) (30.2179, 34.5431) knots 0 0 0 1 2 2 2
  line L241 (30.2179, 34.5431) -> (30.2475, 34.4917)
  spline S143 degree 2 poles (30.2475, 34.4917) (30.4343, 34.5539) (30.9043, 34.6197) (31.1559, 34.5595) knots 0 0 0 1 2 2 2
  spline S144 degree 2 poles (31.1559, 34.5595) (31.4051, 34.5036) (31.8874, 34.1428) (32.0876, 33.796) knots 0 0 0 1 2 2 2
  spline S145 degree 2 poles (32.0876, 33.796) (32.2928, 33.4407) (32.3972, 32.6962) (32.3081, 32.3365) knots 0 0 0 1 2 2 2
  spline S146 degree 2 poles (32.3081, 32.3365) (32.2153, 31.9633) (31.7037, 31.3368) (31.2884, 31.0971) knots 0 0 0 1 2 2 2
  spline S147 degree 2 poles (31.2884, 31.0971) (30.8903, 30.8672) (29.9999, 30.61) (29.6579, 30.5895) knots 0 0 0 1 2 2 2
  line L242 (29.6579, 30.5895) -> (29.2254, 31.3387)
  line L243 (29.2254, 31.3387) -> (29.2767, 31.3683)
  spline S148 degree 2 poles (29.2767, 31.3683) (29.5933, 31.3342) (30.5197, 31.4695) (30.8922, 31.6845) knots 0 0 0 1 2 2 2
  spline S149 degree 2 poles (30.8922, 31.6845) (31.1105, 31.8106) (31.4681, 32.1997) (31.5222, 32.4421) knots 0 0 0 1 2 2 2
  spline S150 degree 2 poles (31.5222, 32.4421) (31.572, 32.6821) (31.5044, 33.1453) (31.3388, 33.4322) knots 0 0 0 1 2 2 2
  spline S151 degree 2 poles (31.3388, 33.4322) (31.1732, 33.719) (30.7912, 33.995) (30.5795, 34.0156) knots 0 0 0 1 2 2 2
  spline S152 degree 2 poles (30.5795, 34.0156) (30.3679, 34.0361) (29.9143, 33.8826) (29.6745, 33.7442) knots 0 0 0 1 2 2 2
  line L244 (29.6745, 33.7442) -> (29.3748, 33.5712)
  line L245 (29.3748, 33.5712) -> (29.0362, 34.1577)
  line L246 (29.0362, 34.1577) -> (29.2717, 34.2936)
  spline S153 degree 2 poles (29.2717, 34.2936) (29.7469, 34.568) (30.0842, 35.3678) (29.8346, 35.8002) knots 0 0 0 1 2 2 2
  spline S154 degree 2 poles (29.8346, 35.8002) (29.7184, 36.0014) (29.3987, 36.1992) (29.2251, 36.2132) knots 0 0 0 1 2 2 2
  spline S155 degree 2 poles (29.2251, 36.2132) (29.0405, 36.2264) (28.6731, 36.1114) (28.4891, 36.0051) knots 0 0 0 1 2 2 2
  spline S156 degree 2 poles (35.5513, 37.2285) (36.3719, 35.8072) (36.3143, 33.9988) (35.4539, 33.502) knots 0 0 0 1 2 2 2
  spline S157 degree 2 poles (35.4539, 33.502) (34.5805, 32.9978) (32.9794, 33.8828) (32.1761, 35.2741) knots 0 0 0 1 2 2 2
  spline S158 degree 2 poles (32.1761, 35.2741) (31.3505, 36.7039) (31.413, 38.5038) (32.2778, 39.0031) knots 0 0 0 1 2 2 2
  spline S159 degree 2 poles (32.2778, 39.0031) (33.1469, 39.5048) (34.7554, 38.607) (35.5513, 37.2285) knots 0 0 0 1 2 2 2
  spline S160 degree 2 poles (35.5731, 35.0948) (35.525, 35.4153) (35.146, 36.2696) (34.8321, 36.8133) knots 0 0 0 1 2 2 2
  spline S161 degree 2 poles (34.8321, 36.8133) (34.5182, 37.3569) (33.9704, 38.1081) (33.7077, 38.316) knots 0 0 0 1 2 2 2
  spline S162 degree 2 poles (33.7077, 38.316) (33.4449, 38.5239) (32.9118, 38.5871) (32.6164, 38.4166) knots 0 0 0 1 2 2 2
  spline S163 degree 2 poles (32.6164, 38.4166) (32.321, 38.246) (32.1007, 37.7478) (32.15, 37.4053) knots 0 0 0 1 2 2 2
  spline S164 degree 2 poles (32.15, 37.4053) (32.1987, 37.0738) (32.5962, 36.2073) (32.8953, 35.6893) knots 0 0 0 1 2 2 2
  spline S165 degree 2 poles (32.8953, 35.6893) (33.2166, 35.1328) (33.7152, 34.4274) (33.9945, 34.2006) knots 0 0 0 1 2 2 2
  spline S166 degree 2 poles (33.9945, 34.2006) (34.2555, 33.9859) (34.807, 33.9105) (35.1152, 34.0885) knots 0 0 0 1 2 2 2
  spline S167 degree 2 poles (35.1152, 34.0885) (35.4064, 34.2565) (35.6267, 34.7548) (35.5731, 35.0948) knots 0 0 0 1 2 2 2
  spline S168 degree 2 poles (69.3351, 37.1013) (69.1424, 37.2126) (68.707, 37.3384) (68.4809, 37.3719) knots 0 0 0 1 2 2 2
  spline S169 degree 2 poles (68.4809, 37.3719) (68.2677, 37.398) (67.9261, 37.3897) (67.7881, 37.378) knots 0 0 0 1 2 2 2
  line L247 (67.7881, 37.378) -> (67.7453, 37.4027)
  line L248 (67.7453, 37.4027) -> (68.1778, 38.1519)
  spline S170 degree 2 poles (68.1778, 38.1519) (68.4807, 38.1426) (69.3888, 37.8865) (69.7442, 37.6814) knots 0 0 0 1 2 2 2
  spline S171 degree 2 poles (69.7442, 37.6814) (70.1038, 37.4738) (70.5549, 37.0193) (70.6842, 36.7391) knots 0 0 0 1 2 2 2
  spline S172 degree 2 poles (70.6842, 36.7391) (70.819, 36.4387) (70.7794, 35.8165) (70.5916, 35.4912) knots 0 0 0 1 2 2 2
  spline S173 degree 2 poles (70.5916, 35.4912) (70.3395, 35.0545) (69.3852, 34.7264) (68.9334, 34.8731) knots 0 0 0 1 2 2 2
  line L249 (68.9334, 34.8731) -> (68.9037, 34.8218)
  spline S174 degree 2 poles (68.9037, 34.8218) (69.0509, 34.6911) (69.3429, 34.317) (69.4166, 34.069) knots 0 0 0 1 2 2 2
  spline S175 degree 2 poles (69.4166, 34.069) (69.4928, 33.8252) (69.4214, 33.2271) (69.2212, 32.8804) knots 0 0 0 1 2 2 2
  spline S176 degree 2 poles (69.2212, 32.8804) (69.0161, 32.525) (68.4236, 32.0623) (68.0675, 31.9596) knots 0 0 0 1 2 2 2
  spline S177 degree 2 poles (68.0675, 31.9596) (67.6979, 31.8534) (66.8996, 31.9832) (66.4843, 32.223) knots 0 0 0 1 2 2 2
  spline S178 degree 2 poles (66.4843, 32.223) (66.0862, 32.4529) (65.4183, 33.0953) (65.2295, 33.3813) knots 0 0 0 1 2 2 2
  line L250 (65.2295, 33.3813) -> (65.662, 34.1305)
  line L251 (65.662, 34.1305) -> (65.7134, 34.1008)
  spline S179 degree 2 poles (65.7134, 34.1008) (65.8421, 33.8096) (66.4225, 33.0749) (66.7949, 32.8599) knots 0 0 0 1 2 2 2
  spline S180 degree 2 poles (66.7949, 32.8599) (67.0133, 32.7338) (67.529, 32.6187) (67.766, 32.6931) knots 0 0 0 1 2 2 2
  spline S181 degree 2 poles (67.766, 32.6931) (67.9988, 32.7699) (68.3661, 33.0601) (68.5317, 33.347) knots 0 0 0 1 2 2 2
  spline S182 degree 2 poles (68.5317, 33.347) (68.6973, 33.6338) (68.7454, 34.1026) (68.6573, 34.2962) knots 0 0 0 1 2 2 2
  spline S183 degree 2 poles (68.6573, 34.2962) (68.5693, 34.4897) (68.2095, 34.8058) (67.9698, 34.9443) knots 0 0 0 1 2 2 2
  line L252 (67.9698, 34.9443) -> (67.6701, 35.1173)
  line L253 (67.6701, 35.1173) -> (68.0088, 35.7038)
  line L254 (68.0088, 35.7038) -> (68.2442, 35.5678)
  spline S184 degree 2 poles (68.2442, 35.5678) (68.7194, 35.2935) (69.5807, 35.4012) (69.8304, 35.8336) knots 0 0 0 1 2 2 2
  spline S185 degree 2 poles (69.8304, 35.8336) (69.9465, 36.0348) (69.958, 36.4106) (69.8833, 36.5679) knots 0 0 0 1 2 2 2
  spline S186 degree 2 poles (69.8833, 36.5679) (69.8025, 36.7344) (69.5192, 36.9951) (69.3351, 37.1013) knots 0 0 0 1 2 2 2
  spline S187 degree 2 poles (73.9257, 31.5969) (73.1051, 30.1757) (71.5102, 29.3213) (70.6497, 29.8181) knots 0 0 0 1 2 2 2
  spline S188 degree 2 poles (70.6497, 29.8181) (69.7764, 30.3223) (69.7422, 32.1515) (70.5455, 33.5428) knots 0 0 0 1 2 2 2
  spline S189 degree 2 poles (70.5455, 33.5428) (71.371, 34.9726) (72.961, 35.8184) (73.8258, 35.3192) knots 0 0 0 1 2 2 2
  spline S190 degree 2 poles (73.8258, 35.3192) (74.6948, 34.8174) (74.7216, 32.9754) (73.9257, 31.5969) knots 0 0 0 1 2 2 2
  spline S191 degree 2 poles (72.0888, 30.5113) (72.3423, 30.7131) (72.8926, 31.4685) (73.2065, 32.0122) knots 0 0 0 1 2 2 2
  spline S192 degree 2 poles (73.2065, 32.0122) (73.5204, 32.5559) (73.897, 33.4058) (73.9457, 33.7373) knots 0 0 0 1 2 2 2
  spline S193 degree 2 poles (73.9457, 33.7373) (73.9943, 34.0688) (73.7825, 34.5621) (73.4872, 34.7327) knots 0 0 0 1 2 2 2
  spline S194 degree 2 poles (73.4872, 34.7327) (73.1918, 34.9032) (72.6501, 34.8449) (72.3781, 34.6309) knots 0 0 0 1 2 2 2
  spline S195 degree 2 poles (72.3781, 34.6309) (72.1154, 34.423) (71.5638, 33.6456) (71.2647, 33.1276) knots 0 0 0 1 2 2 2
  spline S196 degree 2 poles (71.2647, 33.1276) (70.9434, 32.571) (70.5818, 31.7866) (70.5251, 31.4312) knots 0 0 0 1 2 2 2
  spline S197 degree 2 poles (70.5251, 31.4312) (70.4696, 31.0979) (70.6801, 30.5825) (70.9883, 30.4046) knots 0 0 0 1 2 2 2
  spline S198 degree 2 poles (70.9883, 30.4046) (71.2794, 30.2365) (71.8211, 30.2948) (72.0888, 30.5113) knots 0 0 0 1 2 2 2
  spline S199 degree 2 poles (82.8665, 18.7538) (82.4598, 18.5189) (81.6148, 18.3907) (81.2527, 18.4841) knots 0 0 0 1 2 2 2
  spline S200 degree 2 poles (81.2527, 18.4841) (80.8727, 18.5787) (80.279, 19.0237) (80.0739, 19.379) knots 0 0 0 1 2 2 2
  spline S201 degree 2 poles (80.0739, 19.379) (79.8687, 19.7343) (79.7699, 20.4592) (79.8811, 20.8202) knots 0 0 0 1 2 2 2
  spline S202 degree 2 poles (79.8811, 20.8202) (80.0097, 21.2598) (80.795, 22.1242) (81.4971, 22.5295) knots 0 0 0 1 2 2 2
  spline S203 degree 2 poles (81.4971, 22.5295) (82.1863, 22.9275) (83.4582, 23.2851) (84.0397, 23.227) knots 0 0 0 1 2 2 2
  spline S204 degree 2 poles (84.0397, 23.227) (84.6078, 23.1725) (85.5812, 22.5244) (85.9248, 21.9294) knots 0 0 0 1 2 2 2
  spline S205 degree 2 poles (85.9248, 21.9294) (86.0261, 21.7538) (86.1698, 21.4258) (86.1981, 21.288) knots 0 0 0 1 2 2 2
  line L255 (86.1981, 21.288) -> (85.5174, 20.895)
  line L256 (85.5174, 20.895) -> (85.5001, 20.925)
  spline S206 degree 2 poles (85.5001, 20.925) (85.4946, 21.0531) (85.3769, 21.4646) (85.2582, 21.6701) knots 0 0 0 1 2 2 2
  spline S207 degree 2 poles (85.2582, 21.6701) (84.8776, 22.3294) (83.52, 22.6244) (82.6022, 22.1972) knots 0 0 0 1 2 2 2
  spline S208 degree 2 poles (82.6022, 22.1972) (82.9236, 22.046) (83.4227, 21.6264) (83.6056, 21.3096) knots 0 0 0 1 2 2 2
  spline S209 degree 2 poles (83.6056, 21.3096) (83.7835, 21.0013) (83.9263, 20.4673) (83.8838, 20.106) knots 0 0 0 1 2 2 2
  spline S210 degree 2 poles (83.8838, 20.106) (83.8335, 19.6888) (83.3203, 19.0157) (82.8665, 18.7538) knots 0 0 0 1 2 2 2
  spline S211 degree 2 poles (82.4213, 19.4557) (82.7466, 19.6435) (83.0887, 20.0693) (83.1341, 20.3467) knots 0 0 0 1 2 2 2
  spline S212 degree 2 poles (83.1341, 20.3467) (83.1638, 20.5522) (83.0339, 20.9453) (82.9276, 21.1293) knots 0 0 0 1 2 2 2
  spline S213 degree 2 poles (82.9276, 21.1293) (82.7843, 21.3776) (82.365, 21.7578) (82.0928, 21.9031) knots 0 0 0 1 2 2 2
  spline S214 degree 2 poles (82.0928, 21.9031) (82.0132, 21.8629) (81.8627, 21.7874) (81.7514, 21.7231) knots 0 0 0 1 2 2 2
  spline S215 degree 2 poles (81.7514, 21.7231) (81.2035, 21.4068) (80.6549, 20.8047) (80.5733, 20.5407) knots 0 0 0 1 2 2 2
  spline S216 degree 2 poles (80.5733, 20.5407) (80.4929, 20.2944) (80.548, 19.8925) (80.6543, 19.7084) knots 0 0 0 1 2 2 2
  spline S217 degree 2 poles (80.6543, 19.7084) (80.9015, 19.2803) (81.8134, 19.1047) (82.4213, 19.4557) knots 0 0 0 1 2 2 2
  spline S218 degree 2 poles (86.0545, 15.3773) (84.6332, 14.5567) (82.8248, 14.6142) (82.328, 15.4747) knots 0 0 0 1 2 2 2
  spline S219 degree 2 poles (82.328, 15.4747) (81.8238, 16.348) (82.7088, 17.9492) (84.1001, 18.7525) knots 0 0 0 1 2 2 2
  spline S220 degree 2 poles (84.1001, 18.7525) (85.53, 19.578) (87.3298, 19.5155) (87.8291, 18.6508) knots 0 0 0 1 2 2 2
  spline S221 degree 2 poles (87.8291, 18.6508) (88.3309, 17.7817) (87.433, 16.1731) (86.0545, 15.3773) knots 0 0 0 1 2 2 2
  spline S222 degree 2 poles (83.9209, 15.3555) (84.2413, 15.4035) (85.0956, 15.7826) (85.6393, 16.0965) knots 0 0 0 1 2 2 2
  spline S223 degree 2 poles (85.6393, 16.0965) (86.183, 16.4104) (86.9341, 16.9582) (87.142, 17.2209) knots 0 0 0 1 2 2 2
  spline S224 degree 2 poles (87.142, 17.2209) (87.3499, 17.4837) (87.4132, 18.0168) (87.2426, 18.3122) knots 0 0 0 1 2 2 2
  spline S225 degree 2 poles (87.2426, 18.3122) (87.0721, 18.6075) (86.5738, 18.8279) (86.2313, 18.7785) knots 0 0 0 1 2 2 2
  spline S226 degree 2 poles (86.2313, 18.7785) (85.8998, 18.7299) (85.0334, 18.3324) (84.5154, 18.0333) knots 0 0 0 1 2 2 2
  spline S227 degree 2 poles (84.5154, 18.0333) (83.9588, 17.712) (83.2535, 17.2134) (83.0266, 16.934) knots 0 0 0 1 2 2 2
  spline S228 degree 2 poles (83.0266, 16.934) (82.812, 16.6731) (82.7366, 16.1216) (82.9145, 15.8133) knots 0 0 0 1 2 2 2
  spline S229 degree 2 poles (82.9145, 15.8133) (83.0826, 15.5222) (83.5808, 15.3019) (83.9209, 15.3555) knots 0 0 0 1 2 2 2
  line L257 (85.6325, -23.9268) -> (84.1445, -26.504)
  line L258 (84.1445, -26.504) -> (83.6051, -26.1926)
  line L259 (83.6051, -26.1926) -> (84.1588, -25.2336)
  line L260 (84.1588, -25.2336) -> (80.6184, -23.1896)
  line L261 (80.6184, -23.1896) -> (80.0647, -24.1485)
  line L262 (80.0647, -24.1485) -> (79.581, -23.8692)
  spline S230 degree 2 poles (79.581, -23.8692) (79.8949, -23.3255) (79.8833, -22.6338) (79.4749, -22.3524) knots 0 0 0 1 2 2 2
  line L263 (79.4749, -22.3524) -> (79.7913, -21.8045)
  line L264 (79.7913, -21.8045) -> (84.5518, -24.5529)
  line L265 (84.5518, -24.5529) -> (85.0931, -23.6154)
  line L266 (85.0931, -23.6154) -> (85.6325, -23.9268)
  line L267 (88.0744, -19.6972) -> (86.1935, -22.955)
  line L268 (86.1935, -22.955) -> (85.4443, -22.5225)
  spline S231 degree 2 poles (85.4443, -22.5225) (85.3174, -21.9811) (85.0661, -21.0027) (84.9094, -20.5127) knots 0 0 0 1 2 2 2
  spline S232 degree 2 poles (84.9094, -20.5127) (84.5944, -19.526) (84.0527, -18.6253) (83.6289, -18.3806) knots 0 0 0 1 2 2 2
  spline S233 degree 2 poles (83.6289, -18.3806) (83.4063, -18.2521) (82.9933, -18.1963) (82.8146, -18.2586) knots 0 0 0 1 2 2 2
  spline S234 degree 2 poles (82.8146, -18.2586) (82.6358, -18.321) (82.341, -18.5846) (82.2273, -18.7815) knots 0 0 0 1 2 2 2
  spline S235 degree 2 poles (82.2273, -18.7815) (82.1185, -18.9698) (81.9903, -19.4095) (81.9617, -19.627) knots 0 0 0 1 2 2 2
  spline S236 degree 2 poles (81.9617, -19.627) (81.9351, -19.8115) (81.9457, -20.1886) (81.9562, -20.3088) knots 0 0 0 1 2 2 2
  line L269 (81.9562, -20.3088) -> (81.934, -20.3474)
  line L270 (81.934, -20.3474) -> (81.1805, -19.9124)
  spline S237 degree 2 poles (81.1805, -19.9124) (81.1995, -19.6322) (81.4421, -18.7277) (81.6448, -18.3767) knots 0 0 0 1 2 2 2
  spline S238 degree 2 poles (81.6448, -18.3767) (82.0724, -17.6361) (83.3377, -17.2536) (84.0056, -17.6391) knots 0 0 0 1 2 2 2
  spline S239 degree 2 poles (84.0056, -17.6391) (84.3181, -17.8196) (84.7563, -18.2667) (84.9048, -18.5236) knots 0 0 0 1 2 2 2
  spline S240 degree 2 poles (84.9048, -18.5236) (85.0618, -18.7855) (85.3006, -19.42) (85.4003, -19.7515) knots 0 0 0 1 2 2 2
  spline S241 degree 2 poles (85.4003, -19.7515) (85.5714, -20.2955) (85.8784, -21.563) (85.9644, -21.938) knots 0 0 0 1 2 2 2
  line L271 (85.9644, -21.938) -> (87.4623, -19.3437)
  line L272 (87.4623, -19.3437) -> (88.0744, -19.6972)
  spline S242 degree 2 poles (87.7391, -14.178) (89.1604, -14.9986) (90.0148, -16.5935) (89.518, -17.454) knots 0 0 0 1 2 2 2
  spline S243 degree 2 poles (89.518, -17.454) (89.0137, -18.3273) (87.1846, -18.3615) (85.7933, -17.5582) knots 0 0 0 1 2 2 2
  spline S244 degree 2 poles (85.7933, -17.5582) (84.3634, -16.7327) (83.5176, -15.1427) (84.0169, -14.2779) knots 0 0 0 1 2 2 2
  spline S245 degree 2 poles (84.0169, -14.2779) (84.5186, -13.4089) (86.3606, -13.3821) (87.7391, -14.178) knots 0 0 0 1 2 2 2
  spline S246 degree 2 poles (88.8248, -16.0149) (88.6229, -15.7614) (87.8675, -15.2111) (87.3239, -14.8972) knots 0 0 0 1 2 2 2
  spline S247 degree 2 poles (87.3239, -14.8972) (86.7802, -14.5833) (85.9302, -14.2067) (85.5987, -14.1581) knots 0 0 0 1 2 2 2
  spline S248 degree 2 poles (85.5987, -14.1581) (85.2672, -14.1094) (84.7739, -14.3212) (84.6034, -14.6166) knots 0 0 0 1 2 2 2
  spline S249 degree 2 poles (84.6034, -14.6166) (84.4328, -14.9119) (84.4911, -15.4536) (84.7051, -15.7256) knots 0 0 0 1 2 2 2
  spline S250 degree 2 poles (84.7051, -15.7256) (84.913, -15.9883) (85.6905, -16.5399) (86.2085, -16.839) knots 0 0 0 1 2 2 2
  spline S251 degree 2 poles (86.2085, -16.839) (86.765, -17.1603) (87.5495, -17.5219) (87.9048, -17.5786) knots 0 0 0 1 2 2 2
  spline S252 degree 2 poles (87.9048, -17.5786) (88.2381, -17.6341) (88.7535, -17.4236) (88.9315, -17.1154) knots 0 0 0 1 2 2 2
  spline S253 degree 2 poles (88.9315, -17.1154) (89.0995, -16.8243) (89.0412, -16.2826) (88.8248, -16.0149) knots 0 0 0 1 2 2 2
  line L273 (68.5837, -38.0256) -> (66.0065, -39.5135)
  line L274 (66.0065, -39.5135) -> (65.6951, -38.9741)
  line L275 (65.6951, -38.9741) -> (66.654, -38.4204)
  line L276 (66.654, -38.4204) -> (64.61, -34.88)
  line L277 (64.61, -34.88) -> (63.651, -35.4337)
  line L278 (63.651, -35.4337) -> (63.3717, -34.9499)
  spline S254 degree 2 poles (63.3717, -34.9499) (63.9154, -34.636) (64.2512, -34.0312) (64.0383, -33.5833) knots 0 0 0 1 2 2 2
  line L279 (64.0383, -33.5833) -> (64.5862, -33.267)
  line L280 (64.5862, -33.267) -> (67.3347, -38.0274)
  line L281 (67.3347, -38.0274) -> (68.2722, -37.4861)
  line L282 (68.2722, -37.4861) -> (68.5837, -38.0256)
  spline S255 degree 2 poles (71.7888, -33.9376) (72.0087, -34.3186) (72.1404, -35.1102) (72.0562, -35.4784) knots 0 0 0 1 2 2 2
  spline S256 degree 2 poles (72.0562, -35.4784) (71.972, -35.8467) (71.4691, -36.5081) (71.0581, -36.7453) knots 0 0 0 1 2 2 2
  spline S257 degree 2 poles (71.0581, -36.7453) (70.6814, -36.9628) (69.8487, -37.221) (69.5023, -37.244) knots 0 0 0 1 2 2 2
  line L283 (69.5023, -37.244) -> (69.0698, -36.4948)
  line L284 (69.0698, -36.4948) -> (69.1212, -36.4652)
  spline S258 degree 2 poles (69.1212, -36.4652) (69.2371, -36.4781) (69.6301, -36.4568) (69.8537, -36.419) knots 0 0 0 1 2 2 2
  spline S259 degree 2 poles (69.8537, -36.419) (70.1055, -36.3706) (70.4992, -36.2518) (70.7175, -36.1257) knots 0 0 0 1 2 2 2
  spline S260 degree 2 poles (70.7175, -36.1257) (70.9316, -36.0021) (71.245, -35.6157) (71.2942, -35.3647) knots 0 0 0 1 2 2 2
  spline S261 degree 2 poles (71.2942, -35.3647) (71.3354, -35.1297) (71.2302, -34.6311) (71.0671, -34.3485) knots 0 0 0 1 2 2 2
  spline S262 degree 2 poles (71.0671, -34.3485) (70.9039, -34.066) (70.5422, -33.7953) (70.3275, -33.7595) knots 0 0 0 1 2 2 2
  spline S263 degree 2 poles (70.3275, -33.7595) (70.101, -33.7133) (69.5915, -33.859) (69.3218, -34.0148) knots 0 0 0 1 2 2 2